Autodesk Fusion 360 part; units mm, degrees
(part 5 of 8)
  spline S93 degree 5 poles (36.3323, -51.1049) (36.3329, -51.1053) (36.3465, -51.1174) (36.3733, -51.141) (36.4134, -51.1761) (36.4668, -51.2226) (36.5333, -51.2797) (36.6002, -51.3365) (36.6675, -51.3929) (36.7352, -51.4491) (36.8032, -51.5049) (36.8715, -51.5604) (36.9402, -51.6156) (37.0093, -51.6705) (37.0787, -51.725) (37.1484, -51.7793) (37.2184, -51.8333) (37.2888, -51.887) (37.3594, -51.9404) (37.4304, -51.9936) (37.5016, -52.0464) (37.5732, -52.099) (37.6451, -52.1513) (37.7172, -52.2033) (37.7897, -52.255) (37.8624, -52.3065) (37.9354, -52.3577) (38.0086, -52.4087) (38.0822, -52.4593) (38.156, -52.5098) (38.2301, -52.5599) (38.3044, -52.6098) (38.379, -52.6594) (38.4538, -52.7088) (38.5289, -52.758) (38.6043, -52.8068) (38.6799, -52.8555) (38.7558, -52.9039) (38.8318, -52.952) (38.9082, -52.9999) (38.9847, -53.0475) (39.0616, -53.0949) (39.1386, -53.1421) (39.2159, -53.189) (39.2934, -53.2357) (39.3711, -53.2821) (39.449, -53.3283) (39.5272, -53.3742) (39.6056, -53.42) (39.6842, -53.4655) (39.7631, -53.5107) (39.8421, -53.5557) (39.9214, -53.6005) (39.985, -53.6362) (40.0327, -53.6628) (40.0646, -53.6805) (40.0806, -53.6893) knots 0.270845 0.270845 0.270845 0.270845 0.270845 0.270845 0.271429 0.285714 0.3 0.314286 0.328571 0.342857 0.357143 0.371429 0.385714 0.4 0.414286 0.428571 0.442857 0.457143 0.471429 0.485714 0.5 0.514286 0.528571 0.542857 0.557143 0.571429 0.585714 0.6 0.614286 0.628571 0.642857 0.657143 0.671429 0.685714 0.7 0.714286 0.728571 0.742857 0.757143 0.771429 0.785714 0.8 0.814286 0.828571 0.842857 0.857143 0.871429 0.885714 0.9 0.914286 0.928571 0.942857 0.957143 0.971429 0.985714 1 1 1 1 1 1
  arc A47 (40.0806, -53.6893) -> (41.2741, -52.7774) centre (0, 0) ccw
  spline S94 degree 5 poles (41.2741, -52.7774) (41.2697, -52.7596) (41.261, -52.7242) (41.2479, -52.6711) (41.2302, -52.6004) (41.2078, -52.5122) (41.1851, -52.4241) (41.1622, -52.3361) (41.1389, -52.2483) (41.1154, -52.1607) (41.0916, -52.0732) (41.0675, -51.9858) (41.0431, -51.8986) (41.0185, -51.8116) (40.9935, -51.7247) (40.9682, -51.638) (40.9427, -51.5514) (40.9168, -51.465) (40.8907, -51.3788) (40.8642, -51.2927) (40.8375, -51.2068) (40.8104, -51.1211) (40.783, -51.0355) (40.7554, -50.9502) (40.7274, -50.865) (40.6991, -50.78) (40.6705, -50.6951) (40.6415, -50.6105) (40.6123, -50.526) (40.5827, -50.4417) (40.5528, -50.3577) (40.5226, -50.2738) (40.492, -50.1901) (40.4611, -50.1066) (40.4299, -50.0233) (40.3983, -49.9403) (40.3664, -49.8574) (40.3341, -49.7748) (40.3015, -49.6923) (40.2685, -49.6101) (40.2352, -49.5281) (40.2015, -49.4464) (40.1674, -49.3649) (40.133, -49.2836) (40.0981, -49.2025) (40.0629, -49.1217) (40.0273, -49.0412) (39.9913, -48.9609) (39.955, -48.8809) (39.9181, -48.8011) (39.8809, -48.7217) (39.8433, -48.6425) (39.8125, -48.5787) (39.7892, -48.5308) (39.7734, -48.4988) (39.7654, -48.4825) (39.765, -48.4818) knots -1 -1 -1 -1 -1 -1 -0.985714 -0.971429 -0.957143 -0.942857 -0.928571 -0.914286 -0.9 -0.885714 -0.871429 -0.857143 -0.842857 -0.828571 -0.814286 -0.8 -0.785714 -0.771429 -0.757143 -0.742857 -0.728571 -0.714286 -0.7 -0.685714 -0.671429 -0.657143 -0.642857 -0.628571 -0.614286 -0.6 -0.585714 -0.571429 -0.557143 -0.542857 -0.528571 -0.514286 -0.5 -0.485714 -0.471429 -0.457143 -0.442857 -0.428571 -0.414286 -0.4 -0.385714 -0.371429 -0.357143 -0.342857 -0.328571 -0.314286 -0.3 -0.285714 -0.271429 -0.270845 -0.270845 -0.270845 -0.270845 -0.270845 -0.270845
  spline S95 degree 3 poles (39.8171, -48.239) (39.797, -48.2556) (39.7803, -48.2759) (39.7558, -48.3219) (39.7481, -48.347) (39.7435, -48.3915) (39.7442, -48.4103) (39.7509, -48.4472) (39.7568, -48.465) (39.765, -48.4818) knots 0 0 0 0 0.007813 0.007813 0.015626 0.015626 0.021241 0.021241 0.026855 0.026855 0.026855 0.026855
  arc A48 (39.8171, -48.239) -> (40.847, -47.3701) centre (0, 0) ccw
  spline S96 degree 3 poles (41.0951, -47.3597) (41.074, -47.3444) (41.0501, -47.3334) (40.9995, -47.3211) (40.9732, -47.3199) (40.929, -47.3267) (40.911, -47.3321) (40.877, -47.3477) (40.8612, -47.3579) (40.847, -47.3701) knots 0 0 0 0 0.007813 0.007813 0.015626 0.015626 0.021241 0.021241 0.026855 0.026855 0.026855 0.026855
  spline S97 degree 5 poles (41.0951, -47.3597) (41.0956, -47.3601) (41.1104, -47.3708) (41.1393, -47.3918) (41.1826, -47.4228) (41.2403, -47.4639) (41.312, -47.5143) (41.3841, -47.5644) (41.4565, -47.6141) (41.5292, -47.6634) (41.6023, -47.7124) (41.6757, -47.7611) (41.7494, -47.8094) (41.8234, -47.8573) (41.8978, -47.905) (41.9724, -47.9523) (42.0473, -47.9993) (42.1225, -48.0459) (42.198, -48.0923) (42.2737, -48.1383) (42.3498, -48.184) (42.4261, -48.2294) (42.5027, -48.2745) (42.5795, -48.3194) (42.6566, -48.3639) (42.7339, -48.4081) (42.8115, -48.452) (42.8894, -48.4956) (42.9675, -48.539) (43.0458, -48.582) (43.1244, -48.6248) (43.2032, -48.6673) (43.2822, -48.7095) (43.3615, -48.7514) (43.441, -48.7931) (43.5207, -48.8345) (43.6006, -48.8756) (43.6808, -48.9164) (43.7612, -48.957) (43.8418, -48.9973) (43.9226, -49.0373) (44.0036, -49.0771) (44.0848, -49.1166) (44.1663, -49.1558) (44.2479, -49.1948) (44.3298, -49.2335) (44.4118, -49.272) (44.4941, -49.3102) (44.5765, -49.3481) (44.6591, -49.3858) (44.742, -49.4232) (44.825, -49.4604) (44.9082, -49.4973) (44.9749, -49.5267) (45.0251, -49.5486) (45.0585, -49.5631) (45.0752, -49.5704) knots 0.270845 0.270845 0.270845 0.270845 0.270845 0.270845 0.271429 0.285714 0.3 0.314286 0.328571 0.342857 0.357143 0.371429 0.385714 0.4 0.414286 0.428571 0.442857 0.457143 0.471429 0.485714 0.5 0.514286 0.528571 0.542857 0.557143 0.571429 0.585714 0.6 0.614286 0.628571 0.642857 0.657143 0.671429 0.685714 0.7 0.714286 0.728571 0.742857 0.757143 0.771429 0.785714 0.8 0.814286 0.828571 0.842857 0.857143 0.871429 0.885714 0.9 0.914286 0.928571 0.942857 0.957143 0.971429 0.985714 1 1 1 1 1 1
  arc A49 (45.0752, -49.5704) -> (46.1751, -48.5475) centre (0, 0) ccw
  spline S98 degree 5 poles (46.1751, -48.5475) (46.1691, -48.5302) (46.157, -48.4958) (46.1388, -48.4442) (46.1144, -48.3756) (46.0836, -48.2899) (46.0525, -48.2044) (46.0212, -48.1191) (45.9896, -48.0339) (45.9577, -47.9489) (45.9256, -47.8641) (45.8931, -47.7795) (45.8605, -47.6951) (45.8275, -47.6108) (45.7943, -47.5268) (45.7608, -47.4429) (45.727, -47.3592) (45.6929, -47.2757) (45.6585, -47.1924) (45.6239, -47.1093) (45.589, -47.0264) (45.5538, -46.9437) (45.5183, -46.8612) (45.4825, -46.7789) (45.4464, -46.6968) (45.41, -46.6149) (45.3734, -46.5332) (45.3364, -46.4517) (45.2991, -46.3705) (45.2616, -46.2895) (45.2237, -46.2087) (45.1855, -46.1281) (45.147, -46.0478) (45.1082, -45.9676) (45.0691, -45.8878) (45.0296, -45.8081) (44.9898, -45.7287) (44.9498, -45.6496) (44.9093, -45.5707) (44.8686, -45.492) (44.8275, -45.4137) (44.786, -45.3355) (44.7443, -45.2577) (44.7021, -45.1801) (44.6597, -45.1028) (44.6168, -45.0258) (44.5736, -44.9491) (44.5301, -44.8726) (44.4861, -44.7965) (44.4418, -44.7207) (44.3971, -44.6452) (44.352, -44.57) (44.3152, -44.5095) (44.2873, -44.4641) (44.2686, -44.4337) (44.259, -44.4182) (44.2586, -44.4176) knots -1 -1 -1 -1 -1 -1 -0.985714 -0.971429 -0.957143 -0.942857 -0.928571 -0.914286 -0.9 -0.885714 -0.871429 -0.857143 -0.842857 -0.828571 -0.814286 -0.8 -0.785714 -0.771429 -0.757143 -0.742857 -0.728571 -0.714286 -0.7 -0.685714 -0.671429 -0.657143 -0.642857 -0.628571 -0.614286 -0.6 -0.585714 -0.571429 -0.557143 -0.542857 -0.528571 -0.514286 -0.5 -0.485714 -0.471429 -0.457143 -0.442857 -0.428571 -0.414286 -0.4 -0.385714 -0.371429 -0.357143 -0.342857 -0.328571 -0.314286 -0.3 -0.285714 -0.271429 -0.270845 -0.270845 -0.270845 -0.270845 -0.270845 -0.270845
  spline S99 degree 3 poles (44.2869, -44.1709) (44.2685, -44.1894) (44.2539, -44.2112) (44.2339, -44.2593) (44.2287, -44.2851) (44.2284, -44.3298) (44.231, -44.3485) (44.2411, -44.3845) (44.2487, -44.4017) (44.2586, -44.4176) knots 0 0 0 0 0.007813 0.007813 0.015626 0.015626 0.021241 0.021241 0.026855 0.026855 0.026855 0.026855
  arc A50 (44.2869, -44.1709) -> (45.2282, -43.2067) centre (0, 0) ccw
  spline S100 degree 3 poles (45.4741, -43.1724) (45.4516, -43.1592) (45.4268, -43.1505) (45.3753, -43.1431) (45.349, -43.1445) (45.3056, -43.1555) (45.2882, -43.1626) (45.2559, -43.1815) (45.2411, -43.1931) (45.2282, -43.2067) knots 0 0 0 0 0.007813 0.007813 0.015626 0.015626 0.021241 0.021241 0.026855 0.026855 0.026855 0.026855
  spline S101 degree 5 poles (45.4741, -43.1724) (45.4747, -43.1727) (45.4904, -43.1819) (45.5212, -43.2) (45.5673, -43.2267) (45.6287, -43.262) (45.7049, -43.3053) (45.7815, -43.3482) (45.8584, -43.3907) (45.9355, -43.4328) (46.013, -43.4745) (46.0907, -43.5158) (46.1688, -43.5568) (46.2471, -43.5974) (46.3257, -43.6376) (46.4045, -43.6775) (46.4836, -43.717) (46.563, -43.7562) (46.6426, -43.7951) (46.7224, -43.8336) (46.8025, -43.8717) (46.8828, -43.9096) (46.9634, -43.9471) (47.0442, -43.9843) (47.1252, -44.0211) (47.2065, -44.0577) (47.288, -44.0939) (47.3696, -44.1298) (47.4516, -44.1654) (47.5337, -44.2007) (47.616, -44.2357) (47.6985, -44.2704) (47.7813, -44.3048) (47.8642, -44.3389) (47.9474, -44.3726) (48.0307, -44.4061) (48.1143, -44.4393) (48.198, -44.4722) (48.2819, -44.5049) (48.366, -44.5372) (48.4503, -44.5692) (48.5348, -44.601) (48.6195, -44.6325) (48.7043, -44.6637) (48.7893, -44.6946) (48.8745, -44.7252) (48.9599, -44.7556) (49.0455, -44.7857) (49.1312, -44.8155) (49.2171, -44.845) (49.3031, -44.8743) (49.3893, -44.9033) (49.4757, -44.932) (49.545, -44.9548) (49.597, -44.9717) (49.6317, -44.983) (49.6491, -44.9886) knots 0.270845 0.270845 0.270845 0.270845 0.270845 0.270845 0.271429 0.285714 0.3 0.314286 0.328571 0.342857 0.357143 0.371429 0.385714 0.4 0.414286 0.428571 0.442857 0.457143 0.471429 0.485714 0.5 0.514286 0.528571 0.542857 0.557143 0.571429 0.585714 0.6 0.614286 0.628571 0.642857 0.657143 0.671429 0.685714 0.7 0.714286 0.728571 0.742857 0.757143 0.771429 0.785714 0.8 0.814286 0.828571 0.842857 0.857143 0.871429 0.885714 0.9 0.914286 0.928571 0.942857 0.957143 0.971429 0.985714 1 1 1 1 1 1
  arc A51 (49.6491, -44.9886) -> (50.6451, -43.8643) centre (0, 0) ccw
  spline S102 degree 5 poles (50.6451, -43.8643) (50.6374, -43.8477) (50.6221, -43.8146) (50.599, -43.765) (50.568, -43.699) (50.5291, -43.6168) (50.4899, -43.5347) (50.4505, -43.4528) (50.4108, -43.371) (50.3709, -43.2895) (50.3307, -43.2082) (50.2903, -43.1272) (50.2496, -43.0463) (50.2087, -42.9656) (50.1675, -42.8851) (50.126, -42.8049) (50.0843, -42.7248) (50.0423, -42.645) (50.0001, -42.5654) (49.9576, -42.486) (49.9149, -42.4069) (49.8718, -42.3279) (49.8285, -42.2493) (49.785, -42.1708) (49.7411, -42.0926) (49.697, -42.0146) (49.6527, -41.9368) (49.608, -41.8593) (49.5631, -41.782) (49.5178, -41.705) (49.4723, -41.6282) (49.4266, -41.5517) (49.3805, -41.4755) (49.3341, -41.3995) (49.2875, -41.3238) (49.2405, -41.2483) (49.1933, -41.1731) (49.1457, -41.0982) (49.0979, -41.0236) (49.0497, -40.9492) (49.0013, -40.8752) (48.9525, -40.8014) (48.9034, -40.728) (48.854, -40.6548) (48.8042, -40.582) (48.7542, -40.5094) (48.7038, -40.4372) (48.653, -40.3654) (48.6019, -40.2938) (48.5505, -40.2226) (48.4987, -40.1518) (48.4465, -40.0813) (48.4041, -40.0246) (48.372, -39.9822) (48.3504, -39.9537) (48.3393, -39.9392) (48.3389, -39.9387) knots -1 -1 -1 -1 -1 -1 -0.985714 -0.971429 -0.957143 -0.942857 -0.928571 -0.914286 -0.9 -0.885714 -0.871429 -0.857143 -0.842857 -0.828571 -0.814286 -0.8 -0.785714 -0.771429 -0.757143 -0.742857 -0.728571 -0.714286 -0.7 -0.685714 -0.671429 -0.657143 -0.642857 -0.628571 -0.614286 -0.6 -0.585714 -0.571429 -0.557143 -0.542857 -0.528571 -0.514286 -0.5 -0.485714 -0.471429 -0.457143 -0.442857 -0.428571 -0.414286 -0.4 -0.385714 -0.371429 -0.357143 -0.342857 -0.328571 -0.314286 -0.3 -0.285714 -0.271429 -0.270845 -0.270845 -0.270845 -0.270845 -0.270845 -0.270845
  spline S103 degree 3 poles (48.3433, -39.6904) (48.3268, -39.7105) (48.3143, -39.7337) (48.299, -39.7835) (48.2963, -39.8097) (48.3004, -39.8542) (48.3047, -39.8725) (48.3183, -39.9074) (48.3275, -39.9238) (48.3389, -39.9387) knots 0 0 0 0 0.007813 0.007813 0.015626 0.015626 0.021241 0.021241 0.026855 0.026855 0.026855 0.026855
  arc A52 (48.3433, -39.6904) -> (49.1871, -38.6398) centre (0, 0) ccw
  spline S104 degree 3 poles (49.4285, -38.5819) (49.4049, -38.571) (49.3794, -38.5647) (49.3273, -38.5624) (49.3013, -38.5663) (49.2592, -38.5814) (49.2426, -38.5902) (49.2122, -38.6121) (49.1986, -38.6251) (49.1871, -38.6398) knots 0 0 0 0 0.007813 0.007813 0.015626 0.015626 0.021241 0.021241 0.026855 0.026855 0.026855 0.026855
  spline S105 degree 5 poles (49.4285, -38.5819) (49.4292, -38.5822) (49.4457, -38.5899) (49.4781, -38.6049) (49.5265, -38.6271) (49.591, -38.6563) (49.6711, -38.692) (49.7515, -38.7273) (49.8321, -38.7621) (49.913, -38.7966) (49.9941, -38.8306) (50.0755, -38.8643) (50.1571, -38.8975) (50.2389, -38.9304) (50.321, -38.9628) (50.4034, -38.9949) (50.4859, -39.0266) (50.5687, -39.058) (50.6517, -39.0889) (50.7348, -39.1196) (50.8182, -39.1498) (50.9019, -39.1797) (50.9857, -39.2093) (51.0697, -39.2385) (51.1539, -39.2674) (51.2383, -39.2959) (51.3229, -39.3241) (51.4076, -39.352) (51.4926, -39.3795) (51.5778, -39.4067) (51.6631, -39.4336) (51.7486, -39.4602) (51.8342, -39.4864) (51.9201, -39.5123) (52.0061, -39.5379) (52.0923, -39.5632) (52.1787, -39.5882) (52.2652, -39.6129) (52.3518, -39.6372) (52.4387, -39.6613) (52.5257, -39.685) (52.6128, -39.7085) (52.7001, -39.7317) (52.7876, -39.7545) (52.8752, -39.7771) (52.963, -39.7993) (53.0509, -39.8213) (53.1389, -39.843) (53.2271, -39.8644) (53.3155, -39.8855) (53.404, -39.9063) (53.4926, -39.9269) (53.5813, -39.9471) (53.6524, -39.9631) (53.7058, -39.975) (53.7415, -39.9828) (53.7593, -39.9867) knots 0.270845 0.270845 0.270845 0.270845 0.270845 0.270845 0.271429 0.285714 0.3 0.314286 0.328571 0.342857 0.357143 0.371429 0.385714 0.4 0.414286 0.428571 0.442857 0.457143 0.471429 0.485714 0.5 0.514286 0.528571 0.542857 0.557143 0.571429 0.585714 0.6 0.614286 0.628571 0.642857 0.657143 0.671429 0.685714 0.7 0.714286 0.728571 0.742857 0.757143 0.771429 0.785714 0.8 0.814286 0.828571 0.842857 0.857143 0.871429 0.885714 0.9 0.914286 0.928571 0.942857 0.957143 0.971429 0.985714 1 1 1 1 1 1
  arc A53 (53.7593, -39.9867) -> (54.6422, -38.7716) centre (0, 0) ccw
  spline S106 degree 5 poles (54.6422, -38.7716) (54.6329, -38.7558) (54.6145, -38.7244) (54.5867, -38.6772) (54.5495, -38.6145) (54.5028, -38.5364) (54.4559, -38.4584) (54.4088, -38.3807) (54.3614, -38.3032) (54.3138, -38.226) (54.266, -38.1489) (54.2179, -38.0721) (54.1696, -37.9955) (54.1211, -37.9192) (54.0723, -37.8431) (54.0233, -37.7672) (53.974, -37.6915) (53.9246, -37.6161) (53.8748, -37.541) (53.8249, -37.4661) (53.7747, -37.3914) (53.7242, -37.317) (53.6736, -37.2429) (53.6226, -37.169) (53.5715, -37.0953) (53.52, -37.022) (53.4683, -36.9489) (53.4164, -36.876) (53.3642, -36.8034) (53.3118, -36.7311) (53.2591, -36.6591) (53.2061, -36.5874) (53.1529, -36.5159) (53.0994, -36.4448) (53.0457, -36.3739) (52.9917, -36.3033) (52.9374, -36.2331) (52.8829, -36.1631) (52.828, -36.0934) (52.7729, -36.0241) (52.7175, -35.9551) (52.6619, -35.8864) (52.6059, -35.818) (52.5497, -35.7499) (52.4931, -35.6822) (52.4363, -35.6149) (52.3791, -35.5479) (52.3217, -35.4812) (52.2639, -35.415) (52.2059, -35.3491) (52.1475, -35.2836) (52.0888, -35.2184) (52.0411, -35.1661) (52.005, -35.1269) (51.9807, -35.1007) (51.9683, -35.0874) (51.9679, -35.0869) knots -1 -1 -1 -1 -1 -1 -0.985714 -0.971429 -0.957143 -0.942857 -0.928571 -0.914286 -0.9 -0.885714 -0.871429 -0.857143 -0.842857 -0.828571 -0.814286 -0.8 -0.785714 -0.771429 -0.757143 -0.742857 -0.728571 -0.714286 -0.7 -0.685714 -0.671429 -0.657143 -0.642857 -0.628571 -0.614286 -0.6 -0.585714 -0.571429 -0.557143 -0.542857 -0.528571 -0.514286 -0.5 -0.485714 -0.471429 -0.457143 -0.442857 -0.428571 -0.414286 -0.4 -0.385714 -0.371429 -0.357143 -0.342857 -0.328571 -0.314286 -0.3 -0.285714 -0.271429 -0.270845 -0.270845 -0.270845 -0.270845 -0.270845 -0.270845
  spline S107 degree 3 poles (51.9483, -34.8393) (51.9338, -34.861) (51.9236, -34.8852) (51.9132, -34.9362) (51.913, -34.9625) (51.9214, -35.0065) (51.9275, -35.0243) (51.9444, -35.0577) (51.9551, -35.0731) (51.9679, -35.0869) knots 0 0 0 0 0.007813 0.007813 0.015626 0.015626 0.021241 0.021241 0.026855 0.026855 0.026855 0.026855
  arc A54 (51.9483, -34.8393) -> (52.6867, -33.7122) centre (0, 0) ccw
  spline S108 degree 3 poles (52.9215, -33.6313) (52.8969, -33.6226) (52.8709, -33.6189) (52.8189, -33.6216) (52.7934, -33.628) (52.7529, -33.6471) (52.7372, -33.6574) (52.7091, -33.6821) (52.6968, -33.6964) (52.6867, -33.7122) knots 0 0 0 0 0.007813 0.007813 0.015626 0.015626 0.021241 0.021241 0.026855 0.026855 0.026855 0.026855
  spline S109 degree 5 poles (52.9215, -33.6313) (52.9222, -33.6315) (52.9393, -33.6376) (52.9731, -33.6493) (53.0234, -33.6667) (53.0904, -33.6896) (53.1736, -33.7174) (53.2569, -33.7448) (53.3405, -33.7717) (53.4244, -33.7982) (53.5084, -33.8242) (53.5926, -33.8499) (53.6771, -33.8751) (53.7617, -33.8999) (53.8466, -33.9242) (53.9316, -33.9482) (54.0168, -33.9718) (54.1022, -33.9951) (54.1878, -34.0179) (54.2736, -34.0403) (54.3595, -34.0624) (54.4456, -34.0841) (54.5319, -34.1054) (54.6183, -34.1264) (54.7049, -34.147) (54.7917, -34.1673) (54.8786, -34.1872) (54.9657, -34.2067) (55.0529, -34.2259) (55.1403, -34.2448) (55.2278, -34.2633) (55.3154, -34.2815) (55.4033, -34.2993) (55.4912, -34.3168) (55.5793, -34.334) (55.6675, -34.3509) (55.7559, -34.3674) (55.8444, -34.3836) (55.933, -34.3995) (56.0217, -34.4151) (56.1106, -34.4303) (56.1996, -34.4453) (56.2888, -34.4599) (56.378, -34.4742) (56.4674, -34.4882) (56.5569, -34.5019) (56.6465, -34.5153) (56.7363, -34.5284) (56.8261, -34.5411) (56.9161, -34.5536) (57.0062, -34.5658) (57.0963, -34.5777) (57.1866, -34.5893) (57.259, -34.5983) (57.3133, -34.605) (57.3495, -34.6094) (57.3676, -34.6115) knots 0.270845 0.270845 0.270845 0.270845 0.270845 0.270845 0.271429 0.285714 0.3 0.314286 0.328571 0.342857 0.357143 0.371429 0.385714 0.4 0.414286 0.428571 0.442857 0.457143 0.471429 0.485714 0.5 0.514286 0.528571 0.542857 0.557143 0.571429 0.585714 0.6 0.614286 0.628571 0.642857 0.657143 0.671429 0.685714 0.7 0.714286 0.728571 0.742857 0.757143 0.771429 0.785714 0.8 0.814286 0.828571 0.842857 0.857143 0.871429 0.885714 0.9 0.914286 0.928571 0.942857 0.957143 0.971429 0.985714 1 1 1 1 1 1
  arc A55 (57.3676, -34.6115) -> (58.1291, -33.3168) centre (0, 0) ccw
  spline S110 degree 5 poles (58.1291, -33.3168) (58.1184, -33.302) (58.097, -33.2725) (58.0648, -33.2283) (58.0217, -33.1695) (57.9677, -33.0962) (57.9135, -33.0231) (57.859, -32.9503) (57.8044, -32.8778) (57.7496, -32.8055) (57.6945, -32.7334) (57.6393, -32.6616) (57.5838, -32.59) (57.5281, -32.5187) (57.4722, -32.4477) (57.4161, -32.3769) (57.3598, -32.3063) (57.3033, -32.2361) (57.2466, -32.1661) (57.1896, -32.0963) (57.1324, -32.0269) (57.0751, -31.9577) (57.0174, -31.8888) (56.9596, -31.8201) (56.9016, -31.7518) (56.8433, -31.6837) (56.7848, -31.6159) (56.7261, -31.5484) (56.6671, -31.4812) (56.608, -31.4143) (56.5486, -31.3477) (56.4889, -31.2815) (56.4291, -31.2155) (56.369, -31.1498) (56.3087, -31.0845) (56.2481, -31.0194) (56.1873, -30.9547) (56.1262, -30.8903) (56.0649, -30.8263) (56.0034, -30.7626) (55.9416, -30.6992) (55.8795, -30.6362) (55.8173, -30.5736) (55.7547, -30.5113) (55.6919, -30.4493) (55.6288, -30.3878) (55.5655, -30.3266) (55.5019, -30.2658) (55.438, -30.2054) (55.3738, -30.1455) (55.3094, -30.0859) (55.2447, -30.0267) (55.1921, -29.9793) (55.1525, -29.9437) (55.1258, -29.92) (55.1122, -29.9079) (55.1116, -29.9074) knots -1 -1 -1 -1 -1 -1 -0.985714 -0.971429 -0.957143 -0.942857 -0.928571 -0.914286 -0.9 -0.885714 -0.871429 -0.857143 -0.842857 -0.828571 -0.814286 -0.8 -0.785714 -0.771429 -0.757143 -0.742857 -0.728571 -0.714286 -0.7 -0.685714 -0.671429 -0.657143 -0.642857 -0.628571 -0.614286 -0.6 -0.585714 -0.571429 -0.557143 -0.542857 -0.528571 -0.514286 -0.5 -0.485714 -0.471429 -0.457143 -0.442857 -0.428571 -0.414286 -0.4 -0.385714 -0.371429 -0.357143 -0.342857 -0.328571 -0.314286 -0.3 -0.285714 -0.271429 -0.270845 -0.270845 -0.270845 -0.270845 -0.270845 -0.270845
  spline S111 degree 3 poles (55.0682, -29.663) (55.0559, -29.6859) (55.0481, -29.711) (55.0427, -29.7628) (55.0451, -29.789) (55.0576, -29.8319) (55.0654, -29.8491) (55.0854, -29.8807) (55.0976, -29.895) (55.1116, -29.9074) knots 0 0 0 0 0.007813 0.007813 0.015626 0.015626 0.021241 0.021241 0.026855 0.026855 0.026855 0.026855
  arc A56 (55.0682, -29.663) -> (55.6945, -28.4698) centre (0, 0) ccw
  spline S112 degree 3 poles (55.9203, -28.3666) (55.895, -28.3604) (55.8688, -28.3592) (55.8172, -28.3669) (55.7925, -28.3757) (55.754, -28.3986) (55.7394, -28.4104) (55.7138, -28.4377) (55.703, -28.4531) (55.6945, -28.4698) knots 0 0 0 0 0.007813 0.007813 0.015626 0.015626 0.021241 0.021241 0.026855 0.026855 0.026855 0.026855
  spline S113 degree 5 poles (55.9203, -28.3666) (55.921, -28.3668) (55.9387, -28.3711) (55.9734, -28.3796) (56.0252, -28.3921) (56.0941, -28.4084) (56.1795, -28.428) (56.2651, -28.4472) (56.351, -28.4659) (56.4369, -28.4842) (56.5231, -28.502) (56.6094, -28.5194) (56.6959, -28.5363) (56.7826, -28.5528) (56.8694, -28.5689) (56.9563, -28.5846) (57.0434, -28.5999) (57.1307, -28.6147) (57.218, -28.6292) (57.3056, -28.6433) (57.3932, -28.6569) (57.481, -28.6702) (57.569, -28.6831) (57.657, -28.6957) (57.7452, -28.7078) (57.8335, -28.7196) (57.9219, -28.731) (58.0105, -28.7421) (58.0992, -28.7528) (58.1879, -28.7631) (58.2768, -28.7731) (58.3659, -28.7827) (58.455, -28.792) (58.5442, -28.801) (58.6335, -28.8096) (58.723, -28.8178) (58.8125, -28.8257) (58.9022, -28.8333) (58.9919, -28.8406) (59.0818, -28.8475) (59.1717, -28.8541) (59.2617, -28.8604) (59.3519, -28.8664) (59.4421, -28.872) (59.5324, -28.8773) (59.6228, -28.8823) (59.7133, -28.887) (59.8039, -28.8913) (59.8945, -28.8954) (59.9853, -28.8991) (60.0761, -28.9026) (60.167, -28.9057) (60.258, -28.9085) (60.3309, -28.9105) (60.3856, -28.9119) (60.422, -28.9128) (60.4403, -28.9132) knots 0.270845 0.270845 0.270845 0.270845 0.270845 0.270845 0.271429 0.285714 0.3 0.314286 0.328571 0.342857 0.357143 0.371429 0.385714 0.4 0.414286 0.428571 0.442857 0.457143 0.471429 0.485714 0.5 0.514286 0.528571 0.542857 0.557143 0.571429 0.585714 0.6 0.614286 0.628571 0.642857 0.657143 0.671429 0.685714 0.7 0.714286 0.728571 0.742857 0.757143 0.771429 0.785714 0.8 0.814286 0.828571 0.842857 0.857143 0.871429 0.885714 0.9 0.914286 0.928571 0.942857 0.957143 0.971429 0.985714 1 1 1 1 1 1
  arc A57 (60.4403, -28.9132) -> (61.0732, -27.551) centre (0, 0) ccw
  spline S114 degree 5 poles (61.0732, -27.551) (61.0612, -27.5373) (61.037, -27.51) (61.0007, -27.4691) (60.9522, -27.4147) (60.8913, -27.347) (60.8303, -27.2795) (60.7691, -27.2123) (60.7077, -27.1454) (60.6462, -27.0787) (60.5844, -27.0123) (60.5225, -26.9461) (60.4604, -26.8802) (60.3981, -26.8146) (60.3356, -26.7493) (60.2729, -26.6843) (60.2101, -26.6195) (60.147, -26.555) (60.0838, -26.4908) (60.0204, -26.4269) (59.9568, -26.3633) (59.893, -26.2999) (59.829, -26.2369) (59.7648, -26.1742) (59.7004, -26.1117) (59.6359, -26.0496) (59.5711, -25.9878) (59.5061, -25.9263) (59.441, -25.8651) (59.3756, -25.8042) (59.3101, -25.7437) (59.2443, -25.6835) (59.1784, -25.6236) (59.1122, -25.564) (59.0459, -25.5048) (58.9793, -25.4459) (58.9125, -25.3874) (58.8455, -25.3292) (58.7784, -25.2713) (58.711, -25.2139) (58.6433, -25.1568) (58.5755, -25.1) (58.5075, -25.0437) (58.4392, -24.9877) (58.3707, -24.9321) (58.302, -24.877) (58.233, -24.8222) (58.1638, -24.7678) (58.0944, -24.7139) (58.0248, -24.6604) (57.9549, -24.6073) (57.8848, -24.5547) (57.8279, -24.5125) (57.785, -24.481) (57.7561, -24.4599) (57.7414, -24.4492) (57.7408, -24.4488) knots -1 -1 -1 -1 -1 -1 -0.985714 -0.971429 -0.957143 -0.942857 -0.928571 -0.914286 -0.9 -0.885714 -0.871429 -0.857143 -0.842857 -0.828571 -0.814286 -0.8 -0.785714 -0.771429 -0.757143 -0.742857 -0.728571 -0.714286 -0.7 -0.685714 -0.671429 -0.657143 -0.642857 -0.628571 -0.614286 -0.6 -0.585714 -0.571429 -0.557143 -0.542857 -0.528571 -0.514286 -0.5 -0.485714 -0.471429 -0.457143 -0.442857 -0.428571 -0.414286 -0.4 -0.385714 -0.371429 -0.357143 -0.342857 -0.328571 -0.314286 -0.3 -0.285714 -0.271429 -0.270845 -0.270845 -0.270845 -0.270845 -0.270845 -0.270845
  spline S115 degree 3 poles (57.6741, -24.2096) (57.664, -24.2336) (57.6587, -24.2594) (57.6583, -24.3115) (57.6631, -24.3373) (57.6798, -24.3789) (57.6892, -24.3952) (57.7122, -24.4247) (57.7257, -24.4378) (57.7408, -24.4488) knots 0 0 0 0 0.007813 0.007813 0.015626 0.015626 0.021241 0.021241 0.026855 0.026855 0.026855 0.026855
  arc A58 (57.6741, -24.2096) -> (58.1822, -22.9616) centre (0, 0) ccw
  spline S116 degree 3 poles (58.397, -22.8371) (58.3713, -22.8334) (58.345, -22.8347) (58.2945, -22.8473) (58.2707, -22.8585) (58.2346, -22.885) (58.2212, -22.8982) (58.1983, -22.9278) (58.1891, -22.9442) (58.1822, -22.9616) knots 0 0 0 0 0.007813 0.007813 0.015626 0.015626 0.021241 0.021241 0.026855 0.026855 0.026855 0.026855
  spline S117 degree 5 poles (58.397, -22.8371) (58.3977, -22.8372) (58.4158, -22.8398) (58.4511, -22.8449) (58.5038, -22.8523) (58.574, -22.8619) (58.6609, -22.8732) (58.748, -22.884) (58.8353, -22.8944) (58.9226, -22.9043) (59.0101, -22.9137) (59.0977, -22.9227) (59.1854, -22.9312) (59.2732, -22.9392) (59.3612, -22.9469) (59.4492, -22.9541) (59.5374, -22.9609) (59.6257, -22.9672) (59.714, -22.9732) (59.8025, -22.9788) (59.8911, -22.9839) (59.9798, -22.9887) (60.0685, -22.993) (60.1574, -22.997) (60.2463, -23.0006) (60.3354, -23.0038) (60.4245, -23.0066) (60.5137, -23.0091) (60.603, -23.0112) (60.6923, -23.0129) (60.7818, -23.0142) (60.8713, -23.0152) (60.9609, -23.0159) (61.0506, -23.0162) (61.1403, -23.0161) (61.2302, -23.0157) (61.32, -23.015) (61.41, -23.0139) (61.5, -23.0124) (61.5901, -23.0106) (61.6803, -23.0085) (61.7705, -23.0061) (61.8608, -23.0033) (61.9511, -23.0002) (62.0415, -22.9968) (62.132, -22.993) (62.2225, -22.989) (62.3131, -22.9846) (62.4037, -22.9798) (62.4944, -22.9748) (62.5852, -22.9695) (62.676, -22.9638) (62.7668, -22.9578) (62.8395, -22.9528) (62.8941, -22.9489) (62.9305, -22.9462) (62.9487, -22.9449) knots 0.270845 0.270845 0.270845 0.270845 0.270845 0.270845 0.271429 0.285714 0.3 0.314286 0.328571 0.342857 0.357143 0.371429 0.385714 0.4 0.414286 0.428571 0.442857 0.457143 0.471429 0.485714 0.5 0.514286 0.528571 0.542857 0.557143 0.571429 0.585714 0.6 0.614286 0.628571 0.642857 0.657143 0.671429 0.685714 0.7 0.714286 0.728571 0.742857 0.757143 0.771429 0.785714 0.8 0.814286 0.828571 0.842857 0.857143 0.871429 0.885714 0.9 0.914286 0.928571 0.942857 0.957143 0.971429 0.985714 1 1 1 1 1 1
  arc A59 (62.9487, -22.9449) -> (63.4472, -21.528) centre (0, 0) ccw
  spline S118 degree 5 poles (63.4472, -21.528) (63.4338, -21.5155) (63.4072, -21.4907) (63.3671, -21.4535) (63.3135, -21.404) (63.2464, -21.3425) (63.1792, -21.2812) (63.1118, -21.2202) (63.0442, -21.1595) (62.9765, -21.0991) (62.9086, -21.0389) (62.8406, -20.9791) (62.7724, -20.9195) (62.7041, -20.8602) (62.6356, -20.8012) (62.5669, -20.7425) (62.4981, -20.6841) (62.4292, -20.626) (62.36, -20.5682) (62.2907, -20.5107) (62.2213, -20.4535) (62.1517, -20.3967) (62.0819, -20.3401) (62.012, -20.2839) (61.9419, -20.2279) (61.8716, -20.1723) (61.8012, -20.117) (61.7306, -20.0621) (61.6598, -20.0075) (61.5889, -19.9532) (61.5178, -19.8993) (61.4466, -19.8457) (61.3751, -19.7924) (61.3035, -19.7395) (61.2318, -19.687) (61.1598, -19.6348) (61.0877, -19.583) (61.0155, -19.5315) (60.943, -19.4804) (60.8704, -19.4297) (60.7975, -19.3794) (60.7246, -19.3295) (60.6514, -19.28) (60.578, -19.2309) (60.5045, -19.1822) (60.4308, -19.1339) (60.3569, -19.086) (60.2828, -19.0386) (60.2085, -18.9916) (60.134, -18.9451) (60.0593, -18.899) (59.9844, -18.8534) (59.9237, -18.8169) (59.878, -18.7896) (59.8472, -18.7715) (59.8315, -18.7622) (59.8309, -18.7618) knots -1 -1 -1 -1 -1 -1 -0.985714 -0.971429 -0.957143 -0.942857 -0.928571 -0.914286 -0.9 -0.885714 -0.871429 -0.857143 -0.842857 -0.828571 -0.814286 -0.8 -0.785714 -0.771429 -0.757143 -0.742857 -0.728571 -0.714286 -0.7 -0.685714 -0.671429 -0.657143 -0.642857 -0.628571 -0.614286 -0.6 -0.585714 -0.571429 -0.557143 -0.542857 -0.528571 -0.514286 -0.5 -0.485714 -0.471429 -0.457143 -0.442857 -0.428571 -0.414286 -0.4 -0.385714 -0.371429 -0.357143 -0.342857 -0.328571 -0.314286 -0.3 -0.285714 -0.271429 -0.270845 -0.270845 -0.270845 -0.270845 -0.270845 -0.270845
  spline S119 degree 3 poles (59.7414, -18.5303) (59.7337, -18.5551) (59.7309, -18.5813) (59.7355, -18.6332) (59.7428, -18.6584) (59.7634, -18.6981) (59.7743, -18.7135) (59.8001, -18.7406) (59.8148, -18.7524) (59.8309, -18.7618) knots 0 0 0 0 0.007813 0.007813 0.015626 0.015626 0.021241 0.021241 0.026855 0.026855 0.026855 0.026855
  arc A60 (59.7414, -18.5303) -> (60.1267, -17.239) centre (0, 0) ccw
  spline S120 degree 3 poles (60.3285, -17.0944) (60.3025, -17.0931) (60.2765, -17.097) (60.2274, -17.1144) (60.2048, -17.1278) (60.1715, -17.1577) (60.1594, -17.1721) (60.1395, -17.2038) (60.1318, -17.221) (60.1267, -17.239) knots 0 0 0 0 0.007813 0.007813 0.015626 0.015626 0.021241 0.021241 0.026855 0.026855 0.026855 0.026855
  spline S121 degree 5 poles (60.3285, -17.0944) (60.3292, -17.0944) (60.3474, -17.0953) (60.3831, -17.0969) (60.4363, -17.0992) (60.507, -17.1019) (60.5947, -17.1048) (60.6824, -17.1072) (60.7702, -17.1091) (60.8581, -17.1105) (60.9461, -17.1114) (61.0341, -17.1119) (61.1223, -17.1119) (61.2105, -17.1115) (61.2987, -17.1106) (61.3871, -17.1092) (61.4755, -17.1075) (61.564, -17.1053) (61.6525, -17.1027) (61.7411, -17.0997) (61.8298, -17.0963) (61.9185, -17.0925) (62.0073, -17.0882) (62.0961, -17.0836) (62.185, -17.0786) (62.2739, -17.0732) (62.3629, -17.0674) (62.4519, -17.0612) (62.541, -17.0547) (62.6301, -17.0478) (62.7192, -17.0405) (62.8084, -17.0329) (62.8977, -17.0249) (62.987, -17.0165) (63.0763, -17.0078) (63.1656, -16.9987) (63.255, -16.9893) (63.3445, -16.9795) (63.4339, -16.9694) (63.5234, -16.9589) (63.613, -16.9481) (63.7025, -16.937) (63.7921, -16.9255) (63.8818, -16.9137) (63.9714, -16.9016) (64.0611, -16.8891) (64.1508, -16.8763) (64.2405, -16.8632) (64.3303, -16.8497) (64.4201, -16.836) (64.5099, -16.8219) (64.5997, -16.8075) (64.6895, -16.7928) (64.7614, -16.7808) (64.8153, -16.7716) (64.8513, -16.7654) (64.8693, -16.7623) knots 0.270845 0.270845 0.270845 0.270845 0.270845 0.270845 0.271429 0.285714 0.3 0.314286 0.328571 0.342857 0.357143 0.371429 0.385714 0.4 0.414286 0.428571 0.442857 0.457143 0.471429 0.485714 0.5 0.514286 0.528571 0.542857 0.557143 0.571429 0.585714 0.6 0.614286 0.628571 0.642857 0.657143 0.671429 0.685714 0.7 0.714286 0.728571 0.742857 0.757143 0.771429 0.785714 0.8 0.814286 0.828571 0.842857 0.857143 0.871429 0.885714 0.9 0.914286 0.928571 0.942857 0.957143 0.971429 0.985714 1 1 1 1 1 1
  arc A61 (64.8693, -16.7623) -> (65.2287, -15.3039) centre (0, 0) ccw
  spline S122 degree 5 poles (65.2287, -15.3039) (65.2143, -15.2928) (65.1853, -15.2707) (65.1418, -15.2375) (65.0837, -15.1935) (65.011, -15.1387) (64.9382, -15.0842) (64.8652, -15.03) (64.7921, -14.9761) (64.7189, -14.9225) (64.6455, -14.8691) (64.572, -14.8161) (64.4984, -14.7634) (64.4247, -14.711) (64.3508, -14.6589) (64.2768, -14.6071) (64.2027, -14.5556) (64.1284, -14.5044) (64.054, -14.4536) (63.9795, -14.403) (63.9049, -14.3528) (63.8301, -14.3029) (63.7552, -14.2534) (63.6801, -14.2041) (63.605, -14.1552) (63.5297, -14.1067) (63.4542, -14.0585) (63.3787, -14.0106) (63.303, -13.963) (63.2272, -13.9159) (63.1512, -13.869) (63.0751, -13.8226) (62.9989, -13.7764) (62.9225, -13.7307) (62.846, -13.6853) (62.7694, -13.6403) (62.6926, -13.5957) (62.6157, -13.5515) (62.5386, -13.5076) (62.4614, -13.4642) (62.3841, -13.4212) (62.3066, -13.3785) (62.229, -13.3363) (62.1513, -13.2945) (62.0734, -13.2531) (61.9953, -13.2121) (61.9172, -13.1716) (61.8388, -13.1316) (61.7603, -13.092) (61.6817, -13.0528) (61.6029, -13.0142) (61.524, -12.976) (61.4601, -12.9455) (61.4119, -12.9229) (61.3795, -12.9077) (61.363, -12.9) (61.3624, -12.8997) knots -1 -1 -1 -1 -1 -1 -0.985714 -0.971429 -0.957143 -0.942857 -0.928571 -0.914286 -0.9 -0.885714 -0.871429 -0.857143 -0.842857 -0.828571 -0.814286 -0.8 -0.785714 -0.771429 -0.757143 -0.742857 -0.728571 -0.714286 -0.7 -0.685714 -0.671429 -0.657143 -0.642857 -0.628571 -0.614286 -0.6 -0.585714 -0.571429 -0.557143 -0.542857 -0.528571 -0.514286 -0.5 -0.485714 -0.471429 -0.457143 -0.442857 -0.428571 -0.414286 -0.4 -0.385714 -0.371429 -0.357143 -0.342857 -0.328571 -0.314286 -0.3 -0.285714 -0.271429 -0.270845 -0.270845 -0.270845 -0.270845 -0.270845 -0.270845
  spline S123 degree 3 poles (61.2509, -12.6779) (61.2456, -12.7034) (61.2454, -12.7297) (61.255, -12.7809) (61.2647, -12.8053) (61.2891, -12.8428) (61.3014, -12.857) (61.3296, -12.8816) (61.3454, -12.8919) (61.3624, -12.8997) knots 0 0 0 0 0.007813 0.007813 0.015626 0.015626 0.021241 0.021241 0.026855 0.026855 0.026855 0.026855
  arc A62 (61.2509, -12.6779) -> (61.5098, -11.3555) centre (0, 0) ccw
  spline S124 degree 3 poles (61.6967, -11.192) (61.6707, -11.1933) (61.6452, -11.1996) (61.598, -11.2217) (61.5768, -11.2373) (61.5465, -11.2702) (61.5359, -11.2857) (61.5192, -11.3192) (61.5132, -11.3371) (61.5098, -11.3555) knots 0 0 0 0 0.007813 0.007813 0.015626 0.015626 0.021241 0.021241 0.026855 0.026855 0.026855 0.026855
  spline S125 degree 5 poles (61.6967, -11.192) (61.6974, -11.192) (61.7156, -11.1911) (61.7513, -11.1893) (61.8045, -11.1864) (61.8752, -11.1823) (61.9627, -11.1767) (62.0502, -11.1706) (62.1378, -11.164) (62.2254, -11.157) (62.3131, -11.1494) (62.4007, -11.1414) (62.4885, -11.1329) (62.5762, -11.1239) (62.664, -11.1145) (62.7518, -11.1047) (62.8396, -11.0944) (62.9275, -11.0837) (63.0153, -11.0726) (63.1032, -11.061) (63.1912, -11.049) (63.2791, -11.0367) (63.367, -11.0239) (63.455, -11.0107) (63.543, -10.9971) (63.631, -10.9832) (63.719, -10.9688) (63.807, -10.9541) (63.895, -10.939) (63.983, -10.9235) (64.0711, -10.9077) (64.1591, -10.8915) (64.2472, -10.8749) (64.3352, -10.8579) (64.4233, -10.8406) (64.5114, -10.823) (64.5995, -10.805) (64.6875, -10.7866) (64.7756, -10.7679) (64.8637, -10.7488) (64.9517, -10.7295) (65.0398, -10.7097) (65.1279, -10.6897) (65.2159, -10.6693) (65.304, -10.6485) (65.3921, -10.6275) (65.4801, -10.6061) (65.5682, -10.5843) (65.6562, -10.5623) (65.7442, -10.5399) (65.8323, -10.5173) (65.9203, -10.4943) (66.0083, -10.4709) (66.0787, -10.452) (66.1315, -10.4377) (66.1667, -10.4281) (66.1842, -10.4233) knots 0.270845 0.270845 0.270845 0.270845 0.270845 0.270845 0.271429 0.285714 0.3 0.314286 0.328571 0.342857 0.357143 0.371429 0.385714 0.4 0.414286 0.428571 0.442857 0.457143 0.471429 0.485714 0.5 0.514286 0.528571 0.542857 0.557143 0.571429 0.585714 0.6 0.614286 0.628571 0.642857 0.657143 0.671429 0.685714 0.7 0.714286 0.728571 0.742857 0.757143 0.771429 0.785714 0.8 0.814286 0.828571 0.842857 0.857143 0.871429 0.885714 0.9 0.914286 0.928571 0.942857 0.957143 0.971429 0.985714 1 1 1 1 1 1
  arc A63 (66.1842, -10.4233) -> (66.4013, -8.937) centre (0, 0) ccw
  spline S126 degree 5 poles (66.4013, -8.937) (66.3858, -8.9274) (66.3548, -8.9081) (66.3083, -8.8793) (66.2463, -8.841) (66.1686, -8.7935) (66.0908, -8.7463) (66.013, -8.6994) (65.935, -8.6528) (65.857, -8.6065) (65.7788, -8.5605) (65.7005, -8.5149) (65.6222, -8.4695) (65.5437, -8.4244) (65.4652, -8.3797) (65.3865, -8.3353) (65.3078, -8.2912) (65.2289, -8.2474) (65.15, -8.204) (65.0709, -8.1609) (64.9918, -8.1181) (64.9125, -8.0757) (64.8332, -8.0336) (64.7538, -7.9918) (64.6742, -7.9504) (64.5946, -7.9093) (64.5149, -7.8686) (64.435, -7.8282) (64.3551, -7.7882) (64.2751, -7.7486) (64.1949, -7.7093) (64.1147, -7.6704) (64.0344, -7.6319) (63.954, -7.5937) (63.8734, -7.5559) (63.7928, -7.5185) (63.7121, -7.4815) (63.6313, -7.4449) (63.5503, -7.4087) (63.4693, -7.3729) (63.3882, -7.3376) (63.307, -7.3026) (63.2257, -7.2681) (63.1442, -7.2339) (63.0627, -7.2003) (62.9811, -7.167) (62.8994, -7.1343) (62.8175, -7.102) (62.7356, -7.0701) (62.6535, -7.0388) (62.5714, -7.0079) (62.4891, -6.9775) (62.4226, -6.9534) (62.3725, -6.9354) (62.3388, -6.9235) (62.3216, -6.9174) (62.3209, -6.9172) knots -1 -1 -1 -1 -1 -1 -0.985714 -0.971429 -0.957143 -0.942857 -0.928571 -0.914286 -0.9 -0.885714 -0.871429 -0.857143 -0.842857 -0.828571 -0.814286 -0.8 -0.785714 -0.771429 -0.757143 -0.742857 -0.728571 -0.714286 -0.7 -0.685714 -0.671429 -0.657143 -0.642857 -0.628571 -0.614286 -0.6 -0.585714 -0.571429 -0.557143 -0.542857 -0.528571 -0.514286 -0.5 -0.485714 -0.471429 -0.457143 -0.442857 -0.428571 -0.414286 -0.4 -0.385714 -0.371429 -0.357143 -0.342857 -0.328571 -0.314286 -0.3 -0.285714 -0.271429 -0.270845 -0.270845 -0.270845 -0.270845 -0.270845 -0.270845
  spline S127 degree 3 poles (62.1886, -6.7071) (62.1858, -6.733) (62.1881, -6.7592) (62.2026, -6.8092) (62.2146, -6.8326) (62.2425, -6.8676) (62.2561, -6.8806) (62.2866, -6.9023) (62.3033, -6.911) (62.3209, -6.9172) knots 0 0 0 0 0.007813 0.007813 0.015626 0.015626 0.021241 0.021241 0.026855 0.026855 0.026855 0.026855
  arc A64 (62.1886, -6.7071) -> (62.3186, -5.3659) centre (0, 0) ccw
  spline S128 degree 3 poles (62.4889, -5.1852) (62.4631, -5.189) (62.4383, -5.1977) (62.3935, -5.2243) (62.3739, -5.2418) (62.347, -5.2775) (62.3378, -5.294) (62.3244, -5.3289) (62.3202, -5.3473) (62.3186, -5.3659) knots 0 0 0 0 0.007813 0.007813 0.015626 0.015626 0.021241 0.021241 0.026855 0.026855 0.026855 0.026855
  spline S129 degree 5 poles (62.4889, -5.1852) (62.4896, -5.1851) (62.5076, -5.1824) (62.5429, -5.1772) (62.5956, -5.1692) (62.6655, -5.1583) (62.7521, -5.1443) (62.8386, -5.1298) (62.9252, -5.1148) (63.0117, -5.0993) (63.0982, -5.0833) (63.1847, -5.0668) (63.2712, -5.0499) (63.3577, -5.0325) (63.4442, -5.0147) (63.5306, -4.9964) (63.617, -4.9777) (63.7034, -4.9586) (63.7898, -4.939) (63.8762, -4.919) (63.9625, -4.8986) (64.0489, -4.8778) (64.1352, -4.8566) (64.2215, -4.835) (64.3077, -4.813) (64.3939, -4.7906) (64.4802, -4.7679) (64.5663, -4.7447) (64.6525, -4.7212) (64.7386, -4.6973) (64.8247, -4.673) (64.9108, -4.6484) (64.9968, -4.6234) (65.0828, -4.598) (65.1688, -4.5723) (65.2548, -4.5462) (65.3407, -4.5198) (65.4266, -4.493) (65.5125, -4.4659) (65.5983, -4.4384) (65.6841, -4.4106) (65.7698, -4.3825) (65.8555, -4.354) (65.9412, -4.3252) (66.0269, -4.2961) (66.1125, -4.2666) (66.1981, -4.2368) (66.2836, -4.2067) (66.3691, -4.1763) (66.4546, -4.1455) (66.54, -4.1144) (66.6254, -4.083) (66.7107, -4.0513) (66.779, -4.0257) (66.8301, -4.0064) (66.8642, -3.9934) (66.8813, -3.9869) knots 0.270845 0.270845 0.270845 0.270845 0.270845 0.270845 0.271429 0.285714 0.3 0.314286 0.328571 0.342857 0.357143 0.371429 0.385714 0.4 0.414286 0.428571 0.442857 0.457143 0.471429 0.485714 0.5 0.514286 0.528571 0.542857 0.557143 0.571429 0.585714 0.6 0.614286 0.628571 0.642857 0.657143 0.671429 0.685714 0.7 0.714286 0.728571 0.742857 0.757143 0.771429 0.785714 0.8 0.814286 0.828571 0.842857 0.857143 0.871429 0.885714 0.9 0.914286 0.928571 0.942857 0.957143 0.971429 0.985714 1 1 1 1 1 1
  arc A65 (66.8813, -3.9869) -> (66.9538, -2.4867) centre (0, 0) ccw
  spline S130 degree 5 poles (66.9538, -2.4867) (66.9375, -2.4785) (66.9048, -2.4623) (66.8557, -2.4382) (66.7903, -2.4061) (66.7084, -2.3663) (66.6265, -2.3268) (66.5444, -2.2876) (66.4623, -2.2488) (66.3802, -2.2102) (66.2979, -2.172) (66.2156, -2.1341) (66.1333, -2.0965) (66.0508, -2.0592) (65.9683, -2.0223) (65.8858, -1.9857) (65.8031, -1.9494) (65.7204, -1.9134) (65.6376, -1.8778) (65.5548, -1.8425) (65.4719, -1.8076) (65.3889, -1.773) (65.3059, -1.7388) (65.2228, -1.7049) (65.1396, -1.6713) (65.0564, -1.6381) (64.9731, -1.6053) (64.8898, -1.5728) (64.8063, -1.5407) (64.7228, -1.509) (64.6393, -1.4776) (64.5557, -1.4466) (64.472, -1.416) (64.3883, -1.3858) (64.3045, -1.356) (64.2206, -1.3265) (64.1367, -1.2975) (64.0528, -1.2689) (63.9687, -1.2407) (63.8846, -1.2129) (63.8005, -1.1855) (63.7162, -1.1585) (63.632, -1.132) (63.5476, -1.1059) (63.4632, -1.0802) (63.3788, -1.055) (63.2943, -1.0303) (63.2097, -1.006) (63.1251, -0.9823) (63.0404, -0.959) (62.9556, -0.9362) (62.8708, -0.9139) (62.8023, -0.8963) (62.7506, -0.8832) (62.716, -0.8746) (62.6983, -0.8702) (62.6976, -0.8701) knots -1 -1 -1 -1 -1 -1 -0.985714 -0.971429 -0.957143 -0.942857 -0.928571 -0.914286 -0.9 -0.885714 -0.871429 -0.857143 -0.842857 -0.828571 -0.814286 -0.8 -0.785714 -0.771429 -0.757143 -0.742857 -0.728571 -0.714286 -0.7 -0.685714 -0.671429 -0.657143 -0.642857 -0.628571 -0.614286 -0.6 -0.585714 -0.571429 -0.557143 -0.542857 -0.528571 -0.514286 -0.5 -0.485714 -0.471429 -0.457143 -0.442857 -0.428571 -0.414286 -0.4 -0.385714 -0.371429 -0.357143 -0.342857 -0.328571 -0.314286 -0.3 -0.285714 -0.271429 -0.270845 -0.270845 -0.270845 -0.270845 -0.270845 -0.270845
  spline S131 degree 3 poles (62.5456, -0.6738) (62.5453, -0.6998) (62.5501, -0.7256) (62.5694, -0.774) (62.5836, -0.7961) (62.6147, -0.8283) (62.6295, -0.8399) (62.662, -0.8586) (62.6794, -0.8656) (62.6976, -0.8701) knots 0 0 0 0 0.007813 0.007813 0.015626 0.015626 0.021241 0.021241 0.026855 0.026855 0.026855 0.026855
  arc A66 (62.5456, -0.6738) -> (62.5456, 0.6738) centre (0, 0) ccw
  spline S132 degree 3 poles (62.6976, 0.8701) (62.6723, 0.8638) (62.6485, 0.8527) (62.6065, 0.8219) (62.5886, 0.8026) (62.5653, 0.7645) (62.5578, 0.7472) (62.5478, 0.7111) (62.5454, 0.6925) (62.5456, 0.6738) knots 0 0 0 0 0.007813 0.007813 0.015626 0.015626 0.021241 0.021241 0.026855 0.026855 0.026855 0.026855
  spline S133 degree 5 poles (62.6976, 0.8701) (62.6983, 0.8702) (62.716, 0.8746) (62.7506, 0.8832) (62.8023, 0.8963) (62.8708, 0.9139) (62.9556, 0.9362) (63.0404, 0.959) (63.1251, 0.9823) (63.2097, 1.006) (63.2943, 1.0303) (63.3788, 1.055) (63.4632, 1.0802) (63.5476, 1.1059) (63.632, 1.132) (63.7162, 1.1585) (63.8005, 1.1855) (63.8846, 1.2129) (63.9687, 1.2407) (64.0528, 1.2689) (64.1367, 1.2975) (64.2206, 1.3265) (64.3045, 1.356) (64.3883, 1.3858) (64.472, 1.416) (64.5557, 1.4466) (64.6393, 1.4776) (64.7228, 1.509) (64.8063, 1.5407) (64.8898, 1.5728) (64.9731, 1.6053) (65.0564, 1.6381) (65.1396, 1.6713) (65.2228, 1.7049) (65.3059, 1.7388) (65.3889, 1.773) (65.4719, 1.8076) (65.5548, 1.8425) (65.6376, 1.8778) (65.7204, 1.9134) (65.8031, 1.9494) (65.8858, 1.9857) (65.9683, 2.0223) (66.0508, 2.0592) (66.1333, 2.0965) (66.2156, 2.1341) (66.2979, 2.172) (66.3802, 2.2102) (66.4623, 2.2488) (66.5444, 2.2876) (66.6265, 2.3268) (66.7084, 2.3663) (66.7903, 2.4061) (66.8557, 2.4382) (66.9048, 2.4623) (66.9375, 2.4785) (66.9538, 2.4867) knots 0.270845 0.270845 0.270845 0.270845 0.270845 0.270845 0.271429 0.285714 0.3 0.314286 0.328571 0.342857 0.357143 0.371429 0.385714 0.4 0.414286 0.428571 0.442857 0.457143 0.471429 0.485714 0.5 0.514286 0.528571 0.542857 0.557143 0.571429 0.585714 0.6 0.614286 0.628571 0.642857 0.657143 0.671429 0.685714 0.7 0.714286 0.728571 0.742857 0.757143 0.771429 0.785714 0.8 0.814286 0.828571 0.842857 0.857143 0.871429 0.885714 0.9 0.914286 0.928571 0.942857 0.957143 0.971429 0.985714 1 1 1 1 1 1
  arc A67 (66.9538, 2.4867) -> (66.8813, 3.9869) centre (0, 0) ccw
  spline S134 degree 5 poles (66.8813, 3.9869) (66.8642, 3.9934) (66.8301, 4.0064) (66.779, 4.0257) (66.7107, 4.0513) (66.6254, 4.083) (66.54, 4.1144) (66.4546, 4.1455) (66.3691, 4.1763) (66.2836, 4.2067) (66.1981, 4.2368) (66.1125, 4.2666) (66.0269, 4.2961) (65.9412, 4.3252) (65.8555, 4.354) (65.7698, 4.3825) (65.6841, 4.4106) (65.5983, 4.4384) (65.5125, 4.4659) (65.4266, 4.493) (65.3407, 4.5198) (65.2548, 4.5462) (65.1688, 4.5723) (65.0828, 4.598) (64.9968, 4.6234) (64.9108, 4.6484) (64.8247, 4.673) (64.7386, 4.6973) (64.6525, 4.7212) (64.5663, 4.7447) (64.4802, 4.7679) (64.3939, 4.7906) (64.3077, 4.813) (64.2215, 4.835) (64.1352, 4.8566) (64.0489, 4.8778) (63.9625, 4.8986) (63.8762, 4.919) (63.7898, 4.939) (63.7034, 4.9586) (63.617, 4.9777) (63.5306, 4.9964) (63.4442, 5.0147) (63.3577, 5.0325) (63.2712, 5.0499) (63.1847, 5.0668) (63.0982, 5.0833) (63.0117, 5.0993) (62.9252, 5.1148) (62.8386, 5.1298) (62.7521, 5.1443) (62.6655, 5.1583) (62.5956, 5.1692) (62.5429, 5.1772) (62.5076, 5.1824) (62.4896, 5.1851) (62.4889, 5.1852) knots -1 -1 -1 -1 -1 -1 -0.985714 -0.971429 -0.957143 -0.942857 -0.928571 -0.914286 -0.9 -0.885714 -0.871429 -0.857143 -0.842857 -0.828571 -0.814286 -0.8 -0.785714 -0.771429 -0.757143 -0.742857 -0.728571 -0.714286 -0.7 -0.685714 -0.671429 -0.657143 -0.642857 -0.628571 -0.614286 -0.6 -0.585714 -0.571429 -0.557143 -0.542857 -0.528571 -0.514286 -0.5 -0.485714 -0.471429 -0.457143 -0.442857 -0.428571 -0.414286 -0.4 -0.385714 -0.371429 -0.357143 -0.342857 -0.328571 -0.314286 -0.3 -0.285714 -0.271429 -0.270845 -0.270845 -0.270845 -0.270845 -0.270845 -0.270845
  spline S135 degree 3 poles (62.3186, 5.3659) (62.3208, 5.34) (62.3281, 5.3147) (62.352, 5.2684) (62.3683, 5.2478) (62.4023, 5.2187) (62.4182, 5.2087) (62.4523, 5.1932) (62.4704, 5.1879) (62.4889, 5.1852) knots 0 0 0 0 0.007813 0.007813 0.015626 0.015626 0.021241 0.021241 0.026855 0.026855 0.026855 0.026855
  arc A68 (62.3186, 5.3659) -> (62.1886, 6.7071) centre (0, 0) ccw
  spline S136 degree 3 poles (62.3209, 6.9172) (62.2964, 6.9085) (62.2737, 6.8952) (62.2349, 6.8605) (62.219, 6.8395) (62.1994, 6.7993) (62.1936, 6.7814) (62.1872, 6.7445) (62.1866, 6.7257) (62.1886, 6.7071) knots 0 0 0 0 0.007813 0.007813 0.015626 0.015626 0.021241 0.021241 0.026855 0.026855 0.026855 0.026855
  spline S137 degree 5 poles (62.3209, 6.9172) (62.3216, 6.9174) (62.3388, 6.9235) (62.3725, 6.9354) (62.4226, 6.9534) (62.4891, 6.9775) (62.5714, 7.0079) (62.6535, 7.0388) (62.7356, 7.0701) (62.8175, 7.102) (62.8994, 7.1343) (62.9811, 7.167) (63.0627, 7.2003) (63.1442, 7.2339) (63.2257, 7.2681) (63.307, 7.3026) (63.3882, 7.3376) (63.4693, 7.3729) (63.5503, 7.4087) (63.6313, 7.4449) (63.7121, 7.4815) (63.7928, 7.5185) (63.8734, 7.5559) (63.954, 7.5937) (64.0344, 7.6319) (64.1147, 7.6704) (64.1949, 7.7093) (64.2751, 7.7486) (64.3551, 7.7882) (64.435, 7.8282) (64.5149, 7.8686) (64.5946, 7.9093) (64.6742, 7.9504) (64.7538, 7.9918) (64.8332, 8.0336) (64.9125, 8.0757) (64.9918, 8.1181) (65.0709, 8.1609) (65.15, 8.204) (65.2289, 8.2474) (65.3078, 8.2912) (65.3865, 8.3353) (65.4652, 8.3797) (65.5437, 8.4244) (65.6222, 8.4695) (65.7005, 8.5149) (65.7788, 8.5605) (65.857, 8.6065) (65.935, 8.6528) (66.013, 8.6994) (66.0908, 8.7463) (66.1686, 8.7935) (66.2463, 8.841) (66.3083, 8.8793) (66.3548, 8.9081) (66.3858, 8.9274) (66.4013, 8.937) knots 0.270845 0.270845 0.270845 0.270845 0.270845 0.270845 0.271429 0.285714 0.3 0.314286 0.328571 0.342857 0.357143 0.371429 0.385714 0.4 0.414286 0.428571 0.442857 0.457143 0.471429 0.485714 0.5 0.514286 0.528571 0.542857 0.557143 0.571429 0.585714 0.6 0.614286 0.628571 0.642857 0.657143 0.671429 0.685714 0.7 0.714286 0.728571 0.742857 0.757143 0.771429 0.785714 0.8 0.814286 0.828571 0.842857 0.857143 0.871429 0.885714 0.9 0.914286 0.928571 0.942857 0.957143 0.971429 0.985714 1 1 1 1 1 1
  arc A69 (66.4013, 8.937) -> (66.1842, 10.4233) centre (0, 0) ccw
  spline S138 degree 5 poles (66.1842, 10.4233) (66.1667, 10.4281) (66.1315, 10.4377) (66.0787, 10.452) (66.0083, 10.4709) (65.9203, 10.4943) (65.8323, 10.5173) (65.7442, 10.5399) (65.6562, 10.5623) (65.5682, 10.5843) (65.4801, 10.6061) (65.3921, 10.6275) (65.304, 10.6485) (65.2159, 10.6693) (65.1279, 10.6897) (65.0398, 10.7097) (64.9517, 10.7295) (64.8637, 10.7488) (64.7756, 10.7679) (64.6875, 10.7866) (64.5995, 10.805) (64.5114, 10.823) (64.4233, 10.8406) (64.3352, 10.8579) (64.2472, 10.8749) (64.1591, 10.8915) (64.0711, 10.9077) (63.983, 10.9235) (63.895, 10.939) (63.807, 10.9541) (63.719, 10.9688) (63.631, 10.9832) (63.543, 10.9971) (63.455, 11.0107) (63.367, 11.0239) (63.2791, 11.0367) (63.1912, 11.049) (63.1032, 11.061) (63.0153, 11.0726) (62.9275, 11.0837) (62.8396, 11.0944) (62.7518, 11.1047) (62.664, 11.1145) (62.5762, 11.1239) (62.4885, 11.1329) (62.4007, 11.1414) (62.3131, 11.1494) (62.2254, 11.157) (62.1378, 11.164) (62.0502, 11.1706) (61.9627, 11.1767) (61.8752, 11.1823) (61.8045, 11.1864) (61.7513, 11.1893) (61.7156, 11.1911) (61.6974, 11.192) (61.6967, 11.192) knots -1 -1 -1 -1 -1 -1 -0.985714 -0.971429 -0.957143 -0.942857 -0.928571 -0.914286 -0.9 -0.885714 -0.871429 -0.857143 -0.842857 -0.828571 -0.814286 -0.8 -0.785714 -0.771429 -0.757143 -0.742857 -0.728571 -0.714286 -0.7 -0.685714 -0.671429 -0.657143 -0.642857 -0.628571 -0.614286 -0.6 -0.585714 -0.571429 -0.557143 -0.542857 -0.528571 -0.514286 -0.5 -0.485714 -0.471429 -0.457143 -0.442857 -0.428571 -0.414286 -0.4 -0.385714 -0.371429 -0.357143 -0.342857 -0.328571 -0.314286 -0.3 -0.285714 -0.271429 -0.270845 -0.270845 -0.270845 -0.270845 -0.270845 -0.270845
  spline S139 degree 3 poles (61.5098, 11.3555) (61.5145, 11.3299) (61.5242, 11.3054) (61.5524, 11.2616) (61.5706, 11.2427) (61.6073, 11.2171) (61.6241, 11.2086) (61.6595, 11.1965) (61.678, 11.1929) (61.6967, 11.192) knots 0 0 0 0 0.007813 0.007813 0.015626 0.015626 0.021241 0.021241 0.026855 0.026855 0.026855 0.026855
  arc A70 (61.5098, 11.3555) -> (61.2509, 12.6779) centre (0, 0) ccw
  spline S140 degree 3 poles (61.3624, 12.8997) (61.3388, 12.8888) (61.3175, 12.8733) (61.2822, 12.835) (61.2684, 12.8126) (61.2528, 12.7707) (61.2488, 12.7523) (61.2459, 12.715) (61.2471, 12.6962) (61.2509, 12.6779) knots 0 0 0 0 0.007813 0.007813 0.015626 0.015626 0.021241 0.021241 0.026855 0.026855 0.026855 0.026855